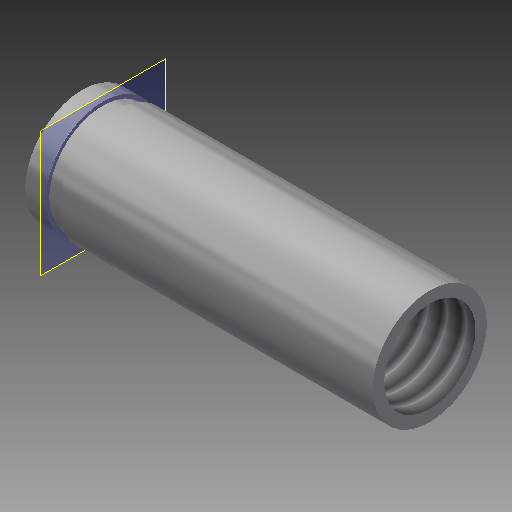
# Autodesk Inventor part: Clutch Sleeve2
Saved by Autodesk Inventor 2017 (Build 210135000, 135)
## iProperties
Created: 2012-08-06
Part Number: Clutch Sleeve2
Material: Steel
Document SubType Name: Modeling
Designer: John
Mass: 2.35773 g
Surface Area: 7.13601 cm^2
Volume: 0.300348 cm^3
Density: 7.85 g/cm^3
Appearance: Steel
Author: John
Autodesk Inventor part; units mm, degrees
ref_plane "YZ Plane" through (0, 0, 0) normal (1, 0, 0) x (0, 1, 0)
ref_plane "XZ Plane" through (0, 0, 0) normal (0, 1, 0) x (-1, 0, 0)
ref_plane "XY Plane" through (0, 0, 0) normal (0, 0, 1) x (1, 0, 0)
sketch "Sketch1" plane through (0, 0, 0) normal (1, 0, 0) x (0, 1, 0)
  circle A0 centre (0, 0) radius 3.175
  dimension "d0" = 6.35
  constraints: 1 centre point, 1 coincident
  measures "d0" diameter of A0
extrude "Extrusion1" add sketch "Sketch1" along normal blind 19.3548
ref_plane "Work Plane1" through (1.143, 0, 0) normal (-1, 0, 0) x (0, 0, 1)
sketch "Sketch2" plane through (1.143, 0, 0) normal (-1, 0, 0) x (0, 0, 1)
  circle A0 centre (0, 0) radius 3.175 projected
  circle A1 centre (0, 0) radius 2.9845
  dimension "d4" = 5.969
  constraints: 1 centre point
  measures "d4" diameter of A1
extrude "Extrusion2" cut sketch "Sketch2" against normal blind 0.762
sketch "Sketch3" plane through (19.3548, 0, 0) normal (1, 0, 0) x (0, 0, -1)
  circle A0 centre (0, 0) radius 3.175 projected
hole "Hole1" at (19.3548, 0, 0) direction (-1, 0, 0) diameter 5.08 depth 14.351
sketch "Sketch4" plane through (0, 0, 0) normal (-1, 0, 0) x (0, 0, 1)
  circle A0 centre (0, 0) radius 3.175 projected
  line L0 (0, 1.2065) -> (1.0449, 0.6033)
  line L1 (1.0449, 0.6033) -> (1.0449, -0.6033)
  line L2 (1.0449, -0.6033) -> (0, -1.2065)
  line L3 (0, -1.2065) -> (-1.0449, -0.6033)
  line L4 (-1.0449, -0.6033) -> (-1.0449, 0.6032)
  line L5 (-1.0449, 0.6032) -> (0, 1.2065)
  dimension "d15" = 2.413
  constraints: 12 end point, 1 coincident, 13 other
  measures "d15" distance of L2.end L0.start
extrude "Extrusion3" cut sketch "Sketch4" against normal through all contours L0 L1 L2 L3 L4 L5
thread "Thread1" size "12-24 UNC" class "2B" standard "ANSI Unified Screw Threads" full length
body "Solid1"
